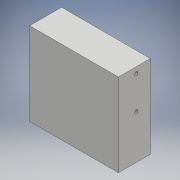
# Autodesk Inventor part: power_supply
Saved by Autodesk Inventor 2018 (Build 220112000, 112)
## iProperties
Created: 2018-02-18
Part Number: power_supply
Material: Generic
Document SubType Name: Modeling
Designer: gaffo
Density: 1 g/cm^3
Appearance: Default
Author: gaffo
Autodesk Inventor part; units mm, degrees
ref_plane "YZ Plane" through (0, 0, 0) normal (1, 0, 0) x (0, 1, 0)
ref_plane "XZ Plane" through (0, 0, 0) normal (0, 1, 0) x (-1, 0, 0)
ref_plane "XY Plane" through (0, 0, 0) normal (0, 0, 1) x (1, 0, 0)
sketch "Sketch1" plane through (0, 0, 0) normal (0, 1, 0) x (-1, 0, 0)
  line L0 (37.5, 35) -> (-37.5, 35)
  line L1 (-37.5, 35) -> (-37.5, -35)
  line L2 (-37.5, -35) -> (37.5, -35)
  line L3 (37.5, -35) -> (37.5, 35)
  point P0 (0, 0)
  point P1 (37.5, 0)
  point P2 (0, -35)
  dimension "d1" = 75
  dimension "d2" = 70
  constraints: 8 end point, 2 midpoint, 2 parallel, 1 horizontal, 1 horizontal alignment, 1 perpendicular, 1 vertical alignment
  measures "d1" distance between parallel lines of L1 L3
  measures "d2" distance between parallel lines of L2 L0
extrude "Extrusion1" add sketch "Sketch1" along normal blind 27
sketch "Sketch2" plane through (37.5, 0, 35) normal (1, 0, 0) x (0, 0, -1)
  circle A0 centre (5, 15) radius 1.5
  line L0 (0, 27) -> (70, 27) projected
  line L1 (0, 0) -> (0, 27) projected
  circle A1 centre (33, 15) radius 1.5
  point P0 (35, 0)
  dimension "d5" = 3
  dimension "d6" = 12
  dimension "d7" = 5
  dimension "d8" = 3
  dimension "d9" = 28
  constraints: 2 centre point
  measures "d5" diameter of A0
  measures "d6" distance from line of A0.centre L0
  measures "d7" distance from line of A0.centre L1
  measures "d8" diameter of A1
  measures "d9" distance of A1.centre A0.centre
extrude "Extrusion2" cut sketch "Sketch2" against normal blind 3
equation "\"d8\" = d5"
body "Solid1"
